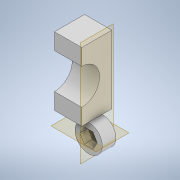
# Autodesk Inventor part: Rear Cable Clamp
Saved by Autodesk Inventor 2020 (Build 240168000, 168)
## iProperties
Created: 2019-12-14
Part Number: Rear Cable Clamp
Material: Generic
Document SubType Name: Modeling
Designer: pepd9
Density: 1 g/cm^3
Appearance: Default
Author: pepd9
Autodesk Inventor part; units mm, degrees
ref_plane "XY Plane" through (0, 0, 0) normal (0, 0, 1) x (1, 0, 0)
sketch "Sketch1" plane through (0, 0, 0) normal (0, 0, 1) x (1, 0, 0)
  circle A0 centre (0, 0) radius 1.7
  circle A1 centre (0, 0) radius 5
  line L0 (0, 7) -> (0, -7) projected
  dimension "d0" = 10
  dimension "d6" = 3.4
  constraints: 2 centre point, 1 coincident
  measures "d0" diameter of A1
  measures "d6" diameter of A0
extrude "Extrusion1" add sketch "Sketch1" along normal blind 5 contours A0 L0 A1 | A0 L0 A1
sketch "Sketch2" plane through (0, 0, 5) normal (0, 0, 1) x (1, 0, 0)
  circle A0 centre (0, 0) radius 1.7 projected
  line L0 (1.5877, 2.75) -> (3.1754, 0)
  line L1 (3.1754, 0) -> (1.5877, -2.75)
  line L2 (1.5877, -2.75) -> (-1.5877, -2.75)
  line L3 (-1.5877, -2.75) -> (-3.1754, 0)
  line L4 (-3.1754, 0) -> (-1.5877, 2.75)
  line L5 (-1.5877, 2.75) -> (1.5877, 2.75)
  dimension "d3" = 5.5
  constraints: 12 end point, 1 coincident, 1 horizontal, 13 other
  measures "d3" distance between parallel lines of L2 L5
extrude "Extrusion2" cut sketch "Sketch2" against normal blind 3
sketch "Sketch3" plane through (0, 0, 0) normal (0, 0, -1) x (-1, 0, 0)
  point P0 (0, 0)
sketch "Sketch4" plane through (0, 0, 0) normal (1, 0, 0) x (0, 1, 0)
  line L0 (5, 0) -> (5, 5) projected
  line L1 (5, -3.5) -> (30, -3.5)
  line L2 (30, -3.5) -> (30, 7.5)
  line L3 (30, 7.5) -> (5, 7.5)
  line L4 (5, 7.5) -> (5, -3.5)
  circle A0 centre (17.5, 7.5) radius 6.5
  line L5 (5, 5) -> (-5, 5) projected
  point P0 (0, 0)
  point P1 (24, 7.5)
  point P2 (11, 7.5)
  dimension "d7" = 13
  dimension "d8" = 25
  dimension "d9" = 12.5
  dimension "d12" = 2.5
  dimension "d13" = 11
  constraints: 8 end point, 2 parallel, 1 centre point, 1 horizontal, 1 midpoint, 1 perpendicular, 1 point on line
  measures "d7" diameter of A0
  measures "d8" distance of L1.start L1.end
  measures "d9" distance from line of L4 A0.centre
  measures "d12" distance between parallel lines of L5 L3
  measures "d13" distance from line of L1 A0.centre
extrude "Extrusion3" add sketch "Sketch4" against normal blind 10 contours L0 L4 L3 A0 L2 L1
body "Solid1"
